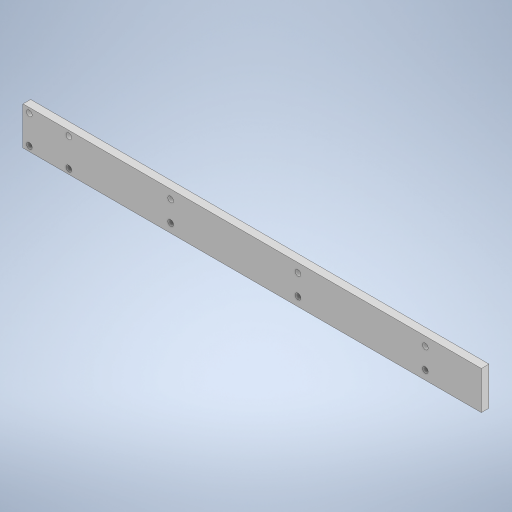
# Autodesk Inventor part: slider_to_cutter_part
Saved by Autodesk Inventor 2024.3 (Build 283343000, 343)
## iProperties
Created: 2025-06-10
Part Number: slider_to_cutter_part
Material: 一般
Document SubType Name: Modeling
Designer: hikou
Density: 1 g/cm^3
Appearance: 既定
Author: hikou
Autodesk Inventor part; units mm, degrees
ref_plane "YZ Plane" through (0, 0, 0) normal (1, 0, 0) x (0, 1, 0)
ref_plane "XZ Plane" through (0, 0, 0) normal (0, 1, 0) x (-1, 0, 0)
ref_plane "XY Plane" through (0, 0, 0) normal (0, 0, 1) x (1, 0, 0)
sketch "スケッチ1" plane through (0, 0, 0) normal (0, 0, 1) x (1, 0, 0)
  line L0 (-90, -7.5) -> (90, -7.5)
  line L1 (90, -7.5) -> (90, 7.5)
  line L2 (90, 7.5) -> (-90, 7.5)
  line L3 (-90, 7.5) -> (-90, -7.5)
  line L4 (-90, -7.5) -> (90, 7.5) construction
  line L5 (90, -7.5) -> (-90, 7.5) construction
  point P0 (0, 0)
  dimension "d0" = 180
  dimension "d1" = 15
  constraints: 12 end point, 2 midpoint, 2 parallel, 1 horizontal, 1 perpendicular
  measures "d0" distance of L1.end L2.end
  measures "d1" distance of L0.end L1.end
extrude "押し出し1" add sketch "スケッチ1" along normal mid plane 3
sketch "スケッチ2" plane through (0, 0, 1.5) normal (0, 0, 1) x (1, 0, 0)
  line L0 (-90, 7.5) -> (-90, -7.5) projected
  line L1 (0, 0) -> (-7.3146, 0)
  point P0 (-87.5, 5.5)
  point P1 (-72, 5.5)
  point P2 (-87.5, -5.5)
  point P3 (-72, -5.5)
  dimension "d4" = 2.5
  dimension "d5" = 15.5
  dimension "d6" = 5.5
  dimension "d7" = 5.5
  constraints: 2 end point, 2 symmetric about line, 1 horizontal
  measures "d4" distance from line of L0 point (-87.5, 5.5)
  measures "d5" distance of point (-72, 5.5) point (-87.5, 5.5)
  measures "d6" vertical distance of L1.start point (-87.5, 5.5)
  measures "d7" vertical distance of L1.start point (-72, 5.5)
hole "穴1" at (-87.5, 5.5, 1.5) at (-72, 5.5, 1.5) at (-87.5, -5.5, 1.5) at (-72, -5.5, 1.5) direction (0, 0, -1) diameter 2.2 end through all
sketch "スケッチ3" plane through (0, 0, 1.5) normal (0, 0, 1) x (1, 0, 0)
  circle A0 centre (-72, 5.5) radius 1.1 projected
  circle A1 centre (-72, -5.5) radius 1.1 projected
  circle A2 centre (-72, -5.5) radius 1.1 projected
  circle A3 centre (-87.5, -5.5) radius 1.1 projected
  circle A4 centre (-72, 5.5) radius 1.1 projected
  circle A5 centre (-87.5, 5.5) radius 1.1 projected
  line L0 (90, -7.5) -> (90, 7.5) projected
  line L1 (90, 7.5) -> (-90, 7.5) projected
  line L2 (-90, 7.5) -> (-90, -7.5) projected
  line L3 (-90, -7.5) -> (90, -7.5) projected
  point P0 (0, 0)
  point P1 (-32, 4)
  point P2 (-32, -4)
  point P3 (18, 4)
  point P4 (18, -4)
  point P5 (68, 4)
  point P6 (68, -4)
  dimension "d15" = 40
  dimension "d16" = 4
  dimension "d17" = 4
  dimension "d18" = 40
  dimension "d28" = 50
  constraints: 1 horizontal, 4 other
  measures "d15" horizontal distance of A0.centre point (-32, 4)
  measures "d16" vertical distance of point (0, 0) point (-32, 4)
  measures "d17" vertical distance of point (0, 0) point (-32, -4)
  measures "d18" horizontal distance of A1.centre point (-32, -4)
  measures "d28" distance of point (-32, 4) point (18, 4)
hole "穴2" at (-32, 4, 1.5) at (-32, -4, 1.5) at (18, 4, 1.5) at (18, -4, 1.5) at (68, 4, 1.5) at (68, -4, 1.5) direction (0, 0, -1) diameter 2.2 end through all
equation "\"d7\" = d6"
equation "\"d17\" = d16"
